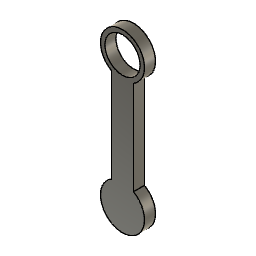
Péndulo v3 (Autodesk Fusion 360 design; units mm, degrees)
Autodesk Fusion 360 part; units mm, degrees
note: some values were not read from the file. Set by a fixed rule: which sketch regions a step uses.
sketch "Boceto1" plane through (0, 0, 0) normal (0, 1, 0) x (1, 0, 0)
  circle A0 centre (0, 0) radius 8
  circle A1 centre (0, 0) radius 10
  line L0 (0, 0) -> (0, 70)
  line L1 (0, 70) -> (0, 60)
  circle A2 centre (0, 60) radius 10
  line L2 (0, 0) -> (-5, 0)
  line L3 (-5, 0) -> (-5, 51.3397)
  line L4 (0, 0) -> (5, 0)
  line L5 (5, 0) -> (5, 51.3397)
  dimension "d1" = 16
  dimension "d2" = 70
  constraint coincident A0.centre A1.centre
  constraint vertical L0
  constraint coincident L0 L1.end
  constraint coincident L1.end A2.centre
  constraint coincident L0.end A2
  constraint perpendicular L0 L2
  constraint coincident A2 L3.end
  constraint perpendicular L2 L3
  constraint perpendicular L0 L4
  constraint coincident A2 L5.end
  constraint perpendicular L4 L5
  measures "d1" diameter of A0
  measures "d2" distance of A0.centre L0.end
extrude "Extruir1" add sketch "Boceto1" along normal blind 5 contours A0 A1 L3 L5 | A0 A1 L0 L5 | A0 A1 L0 L3 | A1 L0 A2 L5 | A1 L0 A2 L3 | L0 L1 A2 | L0 L1 A2
ref_plane "PlanoDeObra1" through (0, 2.5396, -70) normal (0, 0, -1) x (1, 0, 0)
